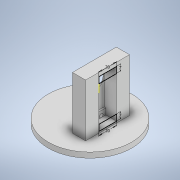
# Autodesk Inventor part: BaseTop
Saved by Autodesk Inventor 2022 (Build 260153000, 153)
## iProperties
Created: 2022-02-03
Part Number: BaseTop
Material: Generic
Document SubType Name: Modeling
Designer: Alexa
Density: 1 g/cm^3
Appearance: Default
Author: Alexa
Autodesk Inventor part; units mm, degrees
ref_plane "YZ Plane" through (0, 0, 0) normal (1, 0, 0) x (0, 1, 0)
ref_plane "XZ Plane" through (0, 0, 0) normal (0, 1, 0) x (-1, 0, 0)
ref_plane "XY Plane" through (0, 0, 0) normal (0, 0, 1) x (1, 0, 0)
sketch "Sketch1" plane through (0, 0, 0) normal (0, 1, 0) x (-1, 0, 0)
  circle A0 centre (0, 0) radius 47.5
  dimension "d0" = 95
  constraints: 1 centre point, 1 coincident
  measures "d0" diameter of A0
extrude "Extrusion1" add sketch "Sketch1" along normal blind 6
sketch "Sketch2" plane through (0, 6, 0) normal (0, 1, 0) x (1, 0, 0)
  circle A0 centre (0, 0) radius 7
  circle A1 centre (0, -7) radius 1.5
  circle A2 centre (0, 7) radius 1.5
  dimension "d3" = 14
  dimension "d4" = 3
  dimension "d5" = 3
  constraints: 3 centre point, 2 point on circle, 1 coincident
  measures "d3" diameter of A0
  measures "d4" diameter of A1
  measures "d5" diameter of A2
extrude "Extrusion2" cut sketch "Sketch2" against normal blind 6 contours A2 A0 | A0 A2 | A1 A0 | A0 A1
sketch "Sketch3" plane through (0, 6, 0) normal (0, 1, 0) x (1, 0, 0)
  line L0 (0, 0) -> (5, 0)
  line L1 (5, 0) -> (5, -10)
  line L2 (5, -10) -> (0, -10)
  line L3 (0, -10) -> (0, 0)
  line L4 (5, 0) -> (0, 0)
  line L5 (0, 0) -> (0, 10)
  line L6 (0, 10) -> (5, 10)
  line L7 (5, 10) -> (5, 0)
  line L8 (5, 0) -> (20, 0)
  line L9 (20, 0) -> (20, -25)
  line L10 (20, -25) -> (5, -25)
  line L11 (5, -25) -> (5, 0)
  line L12 (20, 0) -> (5, 0)
  line L13 (5, 0) -> (5, 25)
  line L14 (5, 25) -> (20, 25)
  line L15 (20, 25) -> (20, 0)
  dimension "d8" = 5
  dimension "d9" = 10
  dimension "d10" = 10
  dimension "d11" = 15
  dimension "d12" = 25
  dimension "d13" = 25
  constraints: 32 end point, 8 parallel, 4 horizontal, 4 perpendicular, 2 point on line
  measures "d8" distance of L1.end L2.end
  measures "d9" distance of L0.end L1.end
  measures "d10" distance of L4.end L5.end
  measures "d11" distance of L9.end L10.end
  measures "d12" distance of L8.end L9.end
  measures "d13" distance of L12.end L13.end
extrude "Extrusion3" add sketch "Sketch3" along normal blind 60 contours L8 L9 L10 L11 L1 | L7 L13 L14 L15 L8
sketch "Sketch4" plane through (5, 6, -25) normal (-1, 0, 0) x (0, 0, 1)
  line L0 (50, 0) -> (50, 60) projected
  line L1 (50, 0) -> (48, 0)
  line L2 (48, 0) -> (48, 40)
  line L3 (48, 40) -> (50, 40)
  line L4 (50, 40) -> (50, 0)
  circle A0 centre (25, 40) radius 10
  point P0 (25, -6)
  dimension "d16" = 2
  dimension "d17" = 40
  dimension "d18" = 20
  constraints: 8 end point, 2 parallel, 1 centre point, 1 horizontal, 1 perpendicular
  measures "d16" distance of L2.end L3.end
  measures "d17" distance of L1.end L2.end
  measures "d18" diameter of A0
extrude "Extrusion4" cut sketch "Sketch4" against normal blind 20 contours A0
sketch "Sketch5" plane through (20, 6, 25) normal (1, 0, 0) x (0, 0, -1)
  circle A0 centre (25, 40) radius 10 projected
  line L0 (25, 40) -> (30, 40)
  line L1 (30, 40) -> (30, 4)
  line L2 (30, 4) -> (25, 4)
  line L3 (25, 4) -> (25, 40)
  line L4 (25, 40) -> (20, 40)
  line L5 (20, 40) -> (20, 4)
  line L6 (20, 4) -> (25, 4)
  line L7 (25, 4) -> (25, 40)
  circle A1 centre (20, 4) radius 2
  circle A2 centre (30, 4) radius 2
  point P0 (25, -6)
  dimension "d21" = 5
  dimension "d22" = 36
  dimension "d23" = 5
  dimension "d24" = 36
  dimension "d25" = 4
  dimension "d26" = 4
  constraints: 16 end point, 4 parallel, 2 centre point, 2 coincident, 2 horizontal, 2 perpendicular
  measures "d21" distance of L1.end L2.end
  measures "d22" distance of L0.end L1.end
  measures "d23" distance of L6.end L5.end
  measures "d24" distance of L5.end L4.end
  measures "d25" diameter of A1
  measures "d26" diameter of A2
extrude "Extrusion5" cut sketch "Sketch5" against normal blind 20 contours A1 L6 L5 | L5 L6 A1 | A2 L2 L1 | L1 L2 A2
sketch "Sketch6" plane through (20, 6, 25) normal (1, 0, 0) x (0, 0, -1)
  line L0 (25, 40) -> (30, 40)
  line L1 (30, 40) -> (30, 54)
  line L2 (30, 54) -> (25, 54)
  line L3 (25, 54) -> (25, 40)
  line L4 (25, 40) -> (20, 40)
  line L5 (20, 40) -> (20, 54)
  line L6 (20, 54) -> (25, 54)
  line L7 (25, 54) -> (25, 40)
  circle A0 centre (20, 54) radius 2
  circle A1 centre (30, 54) radius 2
  point P0 (25, -6)
  dimension "d29" = 5
  dimension "d30" = 14
  dimension "d31" = 5
  dimension "d32" = 14
  dimension "d33" = 4
  dimension "d34" = 4
  constraints: 16 end point, 4 parallel, 2 centre point, 2 coincident, 2 horizontal, 2 perpendicular
  measures "d29" distance of L2.end L1.end
  measures "d30" distance of L1.end L0.end
  measures "d31" distance of L5.end L6.end
  measures "d32" distance of L4.end L5.end
  measures "d33" diameter of A0
  measures "d34" diameter of A1
extrude "Extrusion6" cut sketch "Sketch6" against normal blind 20 contours A1 L2 L1 | L1 L2 A1 | A0 L5 L6 | L6 L5 A0
sketch "Sketch7" plane through (20, 6, 25) normal (1, 0, 0) x (0, 0, -1)
  line L0 (20, 54) -> (30, 54)
  line L1 (30, 54) -> (30, 4)
  line L2 (30, 4) -> (20, 4)
  line L3 (20, 4) -> (20, 54)
  circle A0 centre (20, 54) radius 2 projected
  line L4 (0, 0) -> (0, 60) projected
  line L5 (20, 54) -> (0, 54)
  line L6 (0, 54) -> (0, 49)
  line L7 (0, 49) -> (20, 49)
  line L8 (20, 49) -> (20, 54)
  circle A1 centre (25, 40) radius 10 projected
  line L9 (25, 40) -> (15, 40)
  line L10 (15, 40) -> (15, 30)
  line L11 (15, 30) -> (25, 30)
  line L12 (25, 30) -> (25, 40)
  line L13 (25, 40) -> (35, 40)
  line L14 (35, 40) -> (35, 30)
  line L15 (35, 30) -> (25, 30)
  line L16 (25, 30) -> (25, 40)
  line L17 (35, 40) -> (15, 40)
  line L18 (15, 40) -> (15, 9)
  line L19 (15, 9) -> (35, 9)
  line L20 (35, 9) -> (35, 40)
  line L21 (15, 9) -> (35, 9)
  line L22 (35, 9) -> (35, 49)
  line L23 (35, 49) -> (15, 49)
  line L24 (15, 49) -> (15, 9)
  point P0 (25, -6)
  point P1 (30, 49)
  point P2 (30, 48.6603)
  point P3 (15, 49)
  point P4 (20, 48.6603)
  dimension "d37" = 10
  dimension "d38" = 50
  dimension "d39" = 5
  dimension "d40" = 10
  dimension "d41" = 10
  dimension "d42" = 10
  dimension "d43" = 31
  dimension "d44" = 40
  constraints: 48 end point, 12 parallel, 6 horizontal, 6 perpendicular, 2 point on line
  measures "d37" distance of L1.end L2.end
  measures "d38" distance of L0.end L1.end
  measures "d39" distance of L6.end L5.end
  measures "d40" distance of L11.end L10.end
  measures "d41" distance of L10.end L9.end
  measures "d42" distance of L14.end L15.end
  measures "d43" distance of L18.end L17.end
  measures "d44" distance of L22.end L21.end
extrude "Extrusion7" cut sketch "Sketch7" against normal blind 14 contours L3 A1 L24 L7 | L23 L22 A1 L1 | A1 L3 L11 L10 | L14 L15 L1 A1 | A1 L11 L3 | L11 L3 L19 L18 | L1 L15 A1 | L20 L19 L1 L15 | L11 L15 L1 L19 L3
sketch "Sketch8" plane through (20, 6, 25) normal (1, 0, 0) x (0, 0, -1)
  line L0 (15, 40) -> (15, 49) projected
  line L1 (15, 49) -> (35, 49)
  line L2 (35, 49) -> (35, 56)
  line L3 (35, 56) -> (15, 56)
  line L4 (15, 56) -> (15, 49)
  line L5 (35, 9) -> (15, 9) projected
  line L6 (15, 9) -> (35, 9)
  line L7 (35, 9) -> (35, 2)
  line L8 (35, 2) -> (15, 2)
  line L9 (15, 2) -> (15, 9)
  point P0 (25, -6)
  dimension "d47" = 20
  dimension "d48" = 7
  dimension "d49" = 20
  dimension "d50" = 7
  constraints: 16 end point, 4 parallel, 2 horizontal, 2 perpendicular
  measures "d47" distance of L3.end L2.end
  measures "d48" distance of L2.end L1.end
  measures "d49" distance of L7.end L8.end
  measures "d50" distance of L6.end L7.end
sketch "Sketch9" plane through (20, 6, 25) normal (1, 0, 0) x (0, 0, -1)
  line L0 (15, 40) -> (15, 49) projected
  circle A0 centre (25, 40) radius 10 projected
  line L1 (15, 49) -> (35, 49)
  line L2 (35, 49) -> (35, 40)
  line L3 (35, 40) -> (15, 40)
  line L4 (15, 40) -> (15, 49)
  line L5 (15, 49) -> (20, 49) projected
  line L6 (20, 49) -> (20.777, 49)
  line L7 (20.777, 49) -> (20.777, 48.469)
  line L8 (20.777, 48.469) -> (20, 48.469)
  line L9 (20, 48.469) -> (20, 49)
  line L10 (30, 49) -> (35, 49) projected
  line L11 (30, 49) -> (29.2041, 49)
  line L12 (29.2041, 49) -> (29.2041, 48.469)
  line L13 (29.2041, 48.469) -> (30, 48.469)
  line L14 (30, 48.469) -> (30, 49)
  line L15 (35, 49) -> (35, 9) projected
  line L16 (15, 56) -> (35, 56)
  line L17 (35, 56) -> (35, 49)
  line L18 (35, 49) -> (15, 49)
  line L19 (15, 49) -> (15, 56)
  line L20 (15, 9) -> (15, 49) projected
  line L21 (15, 9) -> (35, 9)
  line L22 (35, 9) -> (35, 2)
  line L23 (35, 2) -> (15, 2)
  line L24 (15, 2) -> (15, 9)
  point P0 (25, -6)
  point P1 (20, 48.6603)
  point P2 (30, 48.6603)
  dimension "d51" = 7
  constraints: 40 end point, 10 parallel, 5 horizontal, 5 perpendicular, 2 point on line, 1 point on circle
  measures "d51" distance of L21.end L22.end
extrude "Extrusion8" cut sketch "Sketch9" against normal blind 12 contours L19 L16 L17 L1 A0 | L9 L1 A0 | L21 L22 L23 L24 | A0 L1 L14
sketch "Sketch10" plane through (8, 60, -5) normal (1, 0, 0) x (0, 0, -1)
  line L0 (-10, -5) -> (-10, -5.3397) projected
  line L1 (-10, -5) -> (0, -5)
  line L2 (0, -5) -> (0, -5.5581)
  line L3 (0, -5.5581) -> (-10, -5.5581)
  line L4 (-10, -5.5581) -> (-10, -5)
  point P0 (-5, -60)
  constraints: 8 end point, 2 parallel, 1 horizontal, 1 perpendicular
extrude "Extrusion9" cut sketch "Sketch10" against normal blind 2
body "Solid1"
